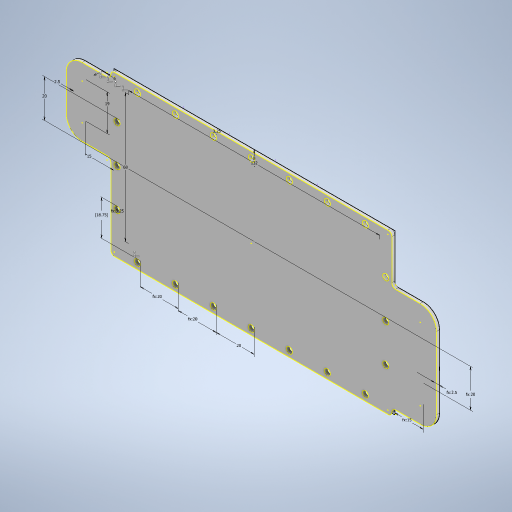
# Autodesk Inventor part: Board Outline
Saved by Autodesk Inventor 2024 (Build 280153000, 153)
## iProperties
Created: 2023-10-10
Part Number: Board Outline
Material: Generic
Document SubType Name: Modeling
Designer: Ishaan
Density: 1 g/cm^3
Appearance: Default
Author: Ishaan
Autodesk Inventor part; units mm, degrees
ref_plane "YZ Plane" through (0, 0, 0) normal (1, 0, 0) x (0, 1, 0)
ref_plane "XZ Plane" through (0, 0, 0) normal (0, 1, 0) x (-1, 0, 0)
ref_plane "XY Plane" through (0, 0, 0) normal (0, 0, 1) x (1, 0, 0)
sketch "Sketch1" plane through (0, 0, 0) normal (0, 0, 1) x (1, 0, 0)
  line L0 (66, -34) -> (-66, -34)
  line L1 (-66, -34) -> (-66, 34)
  line L2 (-66, 34) -> (66, 34)
  line L3 (66, 34) -> (66, -34)
  line L4 (66, -34) -> (-66, 34) construction
  line L5 (-66, -34) -> (66, 34) construction
  line L6 (74, 42) -> (-74, 42)
  line L7 (-74, 42) -> (-74, -42)
  line L8 (-74, -42) -> (74, -42)
  line L9 (74, -42) -> (74, 42)
  line L10 (-74, 38) -> (-89, 38)
  line L11 (-97.5, 29.5) -> (-97.5, 10.5)
  line L12 (-89, 2) -> (-66, 2)
  line L13 (-66, 2) -> (-66, 34)
  line L14 (74, -38) -> (89, -38)
  line L15 (97.5, -29.5) -> (97.5, -10.5)
  line L16 (89, -2) -> (66, -2)
  line L17 (66, -2) -> (66, -34)
  line L18 (-89, 29.5) -> (-89, 10.5) construction
  line L19 (-83, 29.5) -> (-83, 10.5)
  line L20 (-95, 10.5) -> (-95, 29.5)
  arc A0 (-83, 29.5) -> (-95, 29.5) centre (-89, 29.5) ccw
  arc A1 (-95, 10.5) -> (-83, 10.5) centre (-89, 10.5) ccw
  arc A2 (-89, 38) -> (-97.5, 29.5) centre (-89, 29.5) ccw
  arc A3 (-97.5, 10.5) -> (-89, 2) centre (-89, 10.5) ccw
  line L21 (89, -10.5) -> (89, -29.5) construction
  line L22 (83, -10.5) -> (83, -29.5)
  line L23 (95, -29.5) -> (95, -10.5)
  arc A4 (95, -10.5) -> (83, -10.5) centre (89, -10.5) ccw
  arc A5 (83, -29.5) -> (95, -29.5) centre (89, -29.5) ccw
  arc A6 (97.5, -10.5) -> (89, -2) centre (89, -10.5) ccw
  arc A7 (89, -38) -> (97.5, -29.5) centre (89, -29.5) ccw
  line L24 (70.75, -38.75) -> (-70.75, -38.75) construction
  line L25 (-70.75, -38.75) -> (-70.75, 38.75) construction
  line L26 (-70.75, 38.75) -> (70.75, 38.75) construction
  line L27 (70.75, 38.75) -> (70.75, -38.75) construction
  line L28 (70.75, -38.75) -> (-70.75, 38.75) construction
  line L29 (-70.75, -38.75) -> (70.75, 38.75) construction
  line L30 (89, -10.5) -> (89, 8.5) construction
  line L31 (83, -10.5) -> (83, 8.5)
  line L32 (95, 8.5) -> (95, -10.5)
  arc A8 (83, -10.5) -> (95, -10.5) centre (89, -10.5) ccw
  arc A9 (95, 8.5) -> (83, 8.5) centre (89, 8.5) ccw
  line L33 (66, 17) -> (89, 17)
  line L34 (97.5, 8.5) -> (97.5, -10.5)
  arc A10 (97.5, 8.5) -> (89, 17) centre (89, 8.5) ccw
  point P0 (0, 0)
  point P1 (-89, 20)
  point P2 (89, -20)
  point P3 (-74, 2)
  point P4 (74, -38.3314)
  point P5 (74, -2)
  point P6 (-74, 37.5)
  point P7 (-70.75, 20)
  point P8 (-70.75, 0)
  point P9 (-70.75, -20)
  point P10 (-37.446, 41.825)
  point P11 (-13.2416, 41.825)
  point P12 (11.1286, 41.825)
  point P13 (33.3436, 41.825)
  point P14 (70.75, 20)
  point P15 (70.75, 0)
  point P16 (70.75, -20)
  point P17 (-20, -38.75)
  point P18 (-40, -38.75)
  point P19 (-5.5184, 38.75)
  point P20 (-70.75, -13.3991)
  point P21 (70.75, 0)
  point P22 (0, -38.75)
  point P23 (-60, -38.75)
  point P24 (0, -38.75)
  point P25 (89, -1)
  point P26 (74, 17)
  dimension "d0" = 132
  dimension "d1" = 68
  dimension "d2" = 8
  dimension "d5" = 6
  dimension "d6" = 19
  dimension "d8" = 2.5
  dimension "d9" = 15
  dimension "d11" = 2.5
  dimension "d12" = 15
  dimension "d17" = 20
  dimension "d21" = 20
  dimension "d22" = 20
  dimension "d32" = 3.25
  dimension "d33" = 3.25
  dimension "d36" = 20
  dimension "d37" = 20
  dimension "d38" = 18.75
  constraints: 76 end point, 22 point on circle, 22 tangent, 13 parallel, 12 point on line, 11 centre point, 10 midpoint, 9 coincident, 7 perpendicular, 6 horizontal alignment, 4 equal radius, 4 horizontal, 2 equal length, 2 vertical, 1 collinear, 3 other
  measures "d0" distance of L1.end L2.end
  measures "d1" distance of L0.end L1.end
  measures "d2" distance between parallel lines of L2 L6
  measures "d5" radius of A0
  measures "d6" distance of L18.start L18.end
  measures "d8" distance between parallel lines of L20 L11
  measures "d9" distance between parallel lines of L7 L18
  measures "d11" distance between parallel lines of L15 L23
  measures "d12" distance between parallel lines of L9 L21
  measures "d17" distance of point (0, -38.75) point (-20, -38.75)
  measures "d21" distance of point (-20, -38.75) point (-40, -38.75)
  measures "d22" distance of point (-40, -38.75) point (-60, -38.75)
  measures "d32" distance between parallel lines of L26 L6
  measures "d33" distance between parallel lines of L25 L7
  measures "d36" vertical distance of point (0, 0) point (-70.75, 20)
  measures "d37" vertical distance of point (89, -20) point (0, 0)
  measures "d38" vertical distance of point (-70.75, -20) point (-60, -38.75)
extrude "Extrusion1" add sketch "Sketch1" along normal blind 1.6 contours L3 L16 L9 L8 L7 L12 L1 L0 | L0 L1 L2 L3 | L3 L33 L9 L16 | L12 L7 L6 L9 L33 L3 L2 L1 | L16 L31 L22 A5 L23 L32 A6 L15 A7 L14 L9 | L12 A3 L11 A2 L10 L7 | L16 A6 L32 A4 L31 | A8 L23 A5 L22 | A4 A8 | L19 A1 L20 A0
hole "Hole1" at (-70.75, 0, 0) at (-70.75, -20, 0) at (-20, -38.75, 0) at (-40, -38.75, 0) at (0, -38.75, 0) at (-60, -38.75, 0) direction (0, 0, 1) diameter 3.2 end through all
mirror "Mirror1" about plane through (0, 0, 0) normal (1, 0, 0) of "Hole1"
mirror "Mirror2" about plane through (0, 0, 0) normal (0, 1, 0) of "Hole1", "Mirror1"
extrude "Extrusion2" add sketch "Sketch1" along normal up to surface (1.6 mm away) contours L9 L33 A10 L34 A6 L32 A9 L31 L16 | L31 A9 L32 A6 L16
fillet "Fillet1" radius 2 4 edges at (-74, -42, 0.8) (74, -42, 0.8) (74, 42, 0.8) (-74, 42, 0.8)
fillet "Fillet2" radius 2 4 edges at (-74, 2, 0.8) (-74, 38, 0.8) (74, -38, 0.8) (74, 17, 0.8)
sketch "Sketch2" plane through (0, 0, 1.6) normal (0, 0, 1) x (1, 0, 0)
  arc A0 (-72, 42) -> (-74, 40) centre (-72, 40) ccw projected
  line L0 (-74, 0) -> (-74, -40) projected
  arc A1 (-76, 38) -> (-74, 40) centre (-76, 40) ccw projected
  line L1 (-76, 38) -> (-89, 38) projected
  arc A2 (-89, 38) -> (-97.5, 29.5) centre (-89, 29.5) ccw projected
  line L2 (-97.5, 29.5) -> (-97.5, 10.5) projected
  arc A3 (-97.5, 10.5) -> (-89, 2) centre (-89, 10.5) ccw projected
  line L3 (-89, 2) -> (-76, 2) projected
  arc A4 (-74, 0) -> (-76, 2) centre (-76, 0) ccw projected
  arc A5 (-74, -40) -> (-72, -42) centre (-72, -40) ccw projected
  line L4 (-72, -42) -> (72, -42) projected
  arc A6 (72, -42) -> (74, -40) centre (72, -40) ccw projected
  line L5 (74, 19) -> (74, 40) projected
  arc A7 (76, -38) -> (74, -40) centre (76, -40) ccw projected
  line L6 (76, -38) -> (89, -38) projected
  arc A8 (89, -38) -> (97.5, -29.5) centre (89, -29.5) ccw projected
  line L7 (97.5, -29.5) -> (97.5, 8.5) projected
  arc A9 (74, 40) -> (72, 42) centre (72, 40) ccw projected
  line L8 (72, 42) -> (-72, 42) projected
  circle A10 centre (60, 38.75) radius 1.6 projected
  circle A11 centre (70.75, 20) radius 1.6 projected
  circle A12 centre (20, 38.75) radius 1.6 projected
  circle A13 centre (40, 38.75) radius 1.6 projected
  circle A14 centre (-60, 38.75) radius 1.6 projected
  circle A15 centre (-70.75, 20) radius 1.6 projected
  circle A16 centre (-20, 38.75) radius 1.6 projected
  circle A17 centre (-40, 38.75) radius 1.6 projected
  circle A18 centre (0, 38.75) radius 1.6 projected
  circle A19 centre (60, -38.75) radius 1.6 projected
  circle A20 centre (70.75, 0) radius 1.6 projected
  circle A21 centre (70.75, -20) radius 1.6 projected
  circle A22 centre (20, -38.75) radius 1.6 projected
  circle A23 centre (40, -38.75) radius 1.6 projected
  circle A24 centre (-60, -38.75) radius 1.6 projected
  circle A25 centre (0, -38.75) radius 1.6 projected
  circle A26 centre (-40, -38.75) radius 1.6 projected
  circle A27 centre (-20, -38.75) radius 1.6 projected
  circle A28 centre (-70.75, -20) radius 1.6 projected
  circle A29 centre (-70.75, 0) radius 1.6 projected
  arc A30 (97.5, 8.5) -> (89, 17) centre (89, 8.5) ccw projected
  line L9 (76, 17) -> (89, 17) projected
  arc A31 (74, 19) -> (76, 17) centre (76, 19) ccw projected
  point P0 (0, 0)
equation "\"d11\" = d8"
equation "\"d12\" = d9"
equation "\"d21\" = d17"
equation "\"d22\" = d21"
equation "\"d33\" = d32"
equation "\"d37\" = d36"
body "Solid1"
